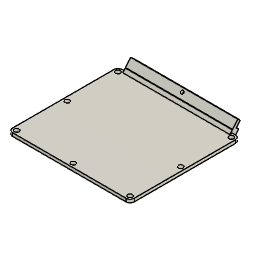
Display Mount Mini - Blank (Autodesk Fusion 360 design; units mm, degrees)
Autodesk Fusion 360 part; units mm, degrees
sketch "Sketch1" plane through (0, 0, 0) normal (0, 0, 1) x (1, 0, 0)
  line L0 (-57.9, 52.128) -> (57.9, 52.128)
  line L1 (57.9, 52.128) -> (57.9, -52.128)
  line L2 (57.9, -52.128) -> (-57.9, -52.128)
  line L3 (-57.9, -52.128) -> (-57.9, 52.128)
  circle A0 centre (-54, 48.228) radius 3.9
  circle A1 centre (-54, 0) radius 2.25
  circle A2 centre (-54, -48.228) radius 3.9
  circle A3 centre (0, -48.228) radius 2.25
  circle A4 centre (54, -48.228) radius 3.9
  circle A5 centre (54, 0) radius 2.25
  circle A6 centre (54, 48.228) radius 3.9
  circle A7 centre (-54, 48.228) radius 2.25
  circle A8 centre (-54, -48.228) radius 2.25
  circle A9 centre (54, -48.228) radius 2.25
  circle A10 centre (54, 48.228) radius 2.25
  point P0 (0, 52.128)
  point P1 (-57.9, 0)
  dimension "d1" = 115.8
  dimension "d2" = 104.256
  dimension "d3" = 7.8
  dimension "d4" = 7.8
  dimension "d5" = 7.8
  dimension "d6" = 7.8
  dimension "d7" = 4.5
  dimension "d8" = 4.5
  dimension "d9" = 4.5
  dimension "d10" = 4.5
  dimension "d11" = 4.5
  dimension "d12" = 4.5
  dimension "d13" = 4.5
  dimension "d14" = 48.128
  dimension "d15" = 96.256
  dimension "d16" = 53.9
  dimension "d17" = 107.8
  constraint horizontal L0
  constraint vertical L1
  constraint horizontal L2
  constraint vertical L3
  constraint midpoint L0 P0
  constraint midpoint L3 P1
  constraint vertical origin P0
  constraint horizontal origin P1
  constraint concentric A0 A7
  constraint concentric A2 A8
  constraint concentric A4 A9
  constraint concentric A6 A10
  constraint tangent L0 A0
  constraint tangent L3 A0
  constraint tangent L1 A4
  constraint tangent L2 A4
  constraint horizontal A0.centre A6.centre
  constraint vertical A5.centre A6.centre
  constraint vertical A5.centre A4.centre
  constraint horizontal A3.centre A2.centre
  constraint horizontal A3.centre A4.centre
  constraint vertical A1.centre A0.centre
  constraint vertical A1.centre A2.centre
  constraint horizontal origin A1.centre
  constraint horizontal origin A5.centre
  constraint vertical origin A3.centre
  measures "d1" distance of L1.end L2.end
  measures "d2" distance of L0.end L1.end
  measures "d3" diameter of A0
  measures "d4" diameter of A2
  measures "d5" diameter of A4
  measures "d6" diameter of A6
  measures "d7" diameter of A1
  measures "d8" diameter of A5
  measures "d9" diameter of A3
  measures "d10" diameter of A7
  measures "d11" diameter of A8
  measures "d12" diameter of A9
  measures "d13" diameter of A10
extrude "Extrude1" add sketch "Sketch1" along normal blind 3 contours L0 L1 L2 L3 A0 A2 A4 A6 | A0 | A6 | A2 | A4
sketch "Sketch2" plane through (0, 0, 0) normal (1, 0, 0) x (0, 1, 0)
  line L0 (-2.25, 3) -> (2.25, 3)
  line L1 (-50.478, 3) -> (-45.978, 3)
  line L2 (-2.25, 3) -> (2.25, 3)
  line L3 (45.978, 3) -> (50.478, 3)
  line L4 (-50.478, 3) -> (-45.978, 3)
  line L5 (45.978, 3) -> (50.478, 3)
  line L6 (-50.478, 3) -> (-45.978, 3)
  line L7 (-48.228, 3) -> (-52.128, 3)
  line L8 (-48.228, 3) -> (48.228, 3)
  line L9 (52.128, 3) -> (48.228, 3)
  line L10 (52.128, 3) -> (48.228, 3)
  line L11 (48.228, 3) -> (-48.228, 3)
  line L12 (-48.228, 3) -> (-52.128, 3)
  line L13 (52.128, 0) -> (52.128, 3)
  line L14 (52.128, 3) -> (52.128, 0)
  line L15 (-2.25, 0) -> (2.25, 0)
  line L16 (-50.478, 0) -> (-45.978, 0)
  line L17 (-2.25, 0) -> (2.25, 0)
  line L18 (45.978, 0) -> (50.478, 0)
  line L19 (-50.478, 0) -> (-45.978, 0)
  line L20 (45.978, 0) -> (50.478, 0)
  line L21 (-50.478, 0) -> (-45.978, 0)
  line L22 (-48.228, 0) -> (-52.128, 0)
  line L23 (-48.228, 0) -> (-52.128, 0)
  line L24 (-48.228, 0) -> (48.228, 0)
  line L25 (52.128, 0) -> (48.228, 0)
  line L26 (52.128, 0) -> (48.228, 0)
  line L27 (48.228, 0) -> (-48.228, 0)
  line L28 (52.128, 3) -> (52.128, 6)
  line L29 (52.128, 6) -> (55.128, 6)
  line L30 (55.128, 6) -> (58.0826, 3.5208)
  line L31 (58.0826, 3.5208) -> (56.1543, 1.2226)
  line L32 (56.1543, 1.2226) -> (62.2826, -3.9197)
  line L33 (62.2826, -3.9197) -> (61.2567, -5.1423)
  line L34 (61.2567, -5.1423) -> (55.1284, 0)
  line L35 (56.1543, 1.2226) -> (55.1284, 0)
  line L36 (55.1284, 0) -> (52.128, 0)
  dimension "d20" = 3
  dimension "d21" = 3
  dimension "d22" = 140
  dimension "d24" = 3.857
  dimension "d26" = 3
  dimension "d27" = 8
  dimension "d28" = 1.596
  constraint coincident L9.start L10.start
  constraint perpendicular L10 L28
  constraint perpendicular L28 L29
  constraint perpendicular L30 L31
  constraint perpendicular L31 L32
  constraint perpendicular L32 L33
  constraint perpendicular L33 L34
  constraint collinear L31 L35
  constraint coincident L13.start L14.end
  measures "d20" distance of L9.start L28.end
  measures "d21" distance of L28.end L29.end
  measures "d22" angle of L29 L30
  measures "d24" distance of L29.end L30.end
  measures "d26" distance of L30.end L31.end
  measures "d27" distance of L31.end L32.end
  measures "d28" distance of L32.end L33.end
extrude "Extrude2" add sketch "Sketch2" along normal mid plane 102 contours L13 L14 L28 L29 L30 L31 L35 L36
sketch "Sketch1 (2)" plane through (0, 25.732, 30.6662) normal (0, 0.642788, 0.766044) x (-1, 0, 0)
  line L0 (51, -38.3738) -> (-51, -38.3738)
  line L1 (-51, -38.3738) -> (-51, -42.2308)
  line L2 (-51, -42.2308) -> (51, -42.2308)
  line L3 (51, -42.2308) -> (51, -38.3738)
  line L4 (51, -39.2308) -> (-51, -39.2308)
  line L5 (-51, -39.2308) -> (-51, -36.2308)
  line L6 (-51, -36.2308) -> (51, -36.2308)
  line L7 (51, -36.2308) -> (51, -39.2308)
  dimension "d67" = 3
  dimension "d68" = 3
  constraint horizontal L4
  constraint vertical L5
  constraint horizontal L6
  constraint vertical L7
  constraint collinear L1 L5
  constraint collinear L3 L7
  measures "d67" distance of L2 L4
  measures "d68" distance of L4 L6
extrude "Extrude4" add sketch "Sketch1 (2)" against normal blind 7 contours L0 L1 L3 L4 L5 L7 | L0 L5 L6 L7
sketch "Sketch2 (2)" plane through (0, 25.732, 30.6662) normal (0, 0.642788, 0.766044) x (-1, 0, 0)
  line L0 (-51, -36.2308) -> (-51, -42.2308)
  line L1 (-51, -42.2308) -> (51, -42.2308)
  line L2 (51, -42.2308) -> (51, -36.2308)
  line L3 (51, -36.2308) -> (-51, -36.2308)
  line L4 (51, -39.2308) -> (-51, -39.2308)
  line L5 (-51, -39.2308) -> (-51, -36.2308)
  line L6 (-51, -36.2308) -> (51, -36.2308)
  line L7 (51, -36.2308) -> (51, -39.2308)
  dimension "d71" = 3
  constraint horizontal L4
  constraint vertical L5
  constraint horizontal L6
  constraint vertical L7
  constraint coincident L0.start L3.end
  constraint coincident L2 L4.start
  measures "d71" distance of L1 L4
extrude "Extrude5" add sketch "Sketch2 (2)" along normal blind 6 contours L0 L2 L3 L4 L5 L6 L7
sketch "Sketch3" plane through (0, 30.0525, -25.2171) normal (0, 0.766044, -0.642788) x (-1, 0, 0)
  line L0 (-51, 40.0319) -> (51, 40.0319)
  line L1 (51, 40.0319) -> (51, 46.0319)
  line L2 (51, 46.0319) -> (-51, 46.0319)
  line L3 (-51, 46.0319) -> (-51, 40.0319)
  circle A0 centre (0, 43.0319) radius 1.425
  dimension "d74" = 2.85
  dimension "d75" = 3
  constraint vertical origin A0.centre
  measures "d74" diameter of A0
  measures "d75" distance of L2 A0.centre
extrude "Extrude6" cut sketch "Sketch3" against normal blind 4 contours A0
equation "d4 = d3"
equation "d5 = d3"
equation "d6 = d3"
equation "d8 = d7"
equation "d9 = d7"
equation "d10 = d7"
equation "d11 = d7"
equation "d12 = d7"
equation "d13 = d7"
